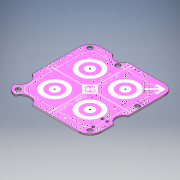
# Autodesk Inventor part: Eagle PCB rev 35
Saved by Autodesk Inventor 2016 (Build 200138000, 138)
## iProperties
Created: 2017-03-15
Part Number: Eagle PCB rev 35
Material: Generic
Document SubType Name: Modeling
Designer: Samuel Clay
Density: 1 g/cm^3
Appearance: Default
Author: Samuel Clay
Autodesk Inventor part; units mm, degrees
(part 1 of 3)
ref_plane "YZ Plane" through (0, 0, 0) normal (1, 0, 0) x (0, 1, 0)
ref_plane "XZ Plane" through (0, 0, 0) normal (0, 1, 0) x (-1, 0, 0)
ref_plane "XY Plane" through (0, 0, 0) normal (0, 0, 1) x (1, 0, 0)
sketch "PCB" plane through (0, 0, 0) normal (0, 0, 1) x (1, 0, 0)
  line L0 (18.3495, -15.3592) -> (18.2813, -15.6127)
  line L1 (15.8202, 13.2003) -> (15.9024, 13.1783)
  line L2 (15.9078, 13.2734) -> (15.9905, 13.2513)
  line L3 (-0.9735, 17.5782) -> (-0.8908, 17.6003)
  line L4 (-1.034, 17.5177) -> (-0.9735, 17.5782)
  line L5 (-1.0562, 17.435) -> (-1.034, 17.5177)
  line L6 (-1.0283, 17.4212) -> (-0.9681, 17.4814)
  line L7 (-0.8908, 17.6003) -> (-0.8082, 17.5782)
  line L8 (-0.8082, 17.5782) -> (-0.7476, 17.5177)
  line L9 (-0.7476, 17.5177) -> (-0.7255, 17.435)
  line L10 (-0.7476, 17.3523) -> (-0.8082, 17.2918)
  line L11 (-0.8082, 17.2918) -> (-0.8908, 17.2697)
  line L12 (-0.8908, 17.2697) -> (-0.9735, 17.2918)
  line L13 (-0.9735, 17.2918) -> (-1.034, 17.3523)
  line L14 (-1.034, 17.3523) -> (-1.0562, 17.435)
  line L15 (-1.034, 17.3523) -> (-1.0283, 17.4212)
  line L16 (-0.9681, 17.4814) -> (-0.8859, 17.5034)
  line L17 (-0.8859, 17.5034) -> (-0.8037, 17.4814)
  line L18 (-0.8037, 17.4814) -> (-0.7435, 17.4212)
  line L19 (-0.7435, 17.4212) -> (-0.7364, 17.3944)
  line L20 (16.6971, -16.0734) -> (16.3265, -16.444)
  line L21 (13.3467, 16.7541) -> (13.4072, 16.8146)
  line L22 (13.4072, 16.8146) -> (13.4899, 16.8368)
  line L23 (13.4899, 16.8368) -> (13.5725, 16.8146)
  line L24 (13.5725, 16.8146) -> (13.633, 16.7541)
  line L25 (13.633, 16.7541) -> (13.6552, 16.6714)
  line L26 (13.6552, 16.6714) -> (13.633, 16.5888)
  line L27 (13.633, 16.5888) -> (13.5725, 16.5282)
  line L28 (13.5725, 16.5282) -> (13.4899, 16.5061)
  line L29 (13.4899, 16.5061) -> (13.4072, 16.5282)
  line L30 (13.4072, 16.5282) -> (13.3467, 16.5888)
  line L31 (13.3467, 16.5888) -> (13.3245, 16.6714)
  line L32 (-7.6358, -7.5426) -> (-7.5426, -7.6358)
  line L33 (1.2213, 5.8377) -> (1.2815, 5.7775)
  line L34 (5.3008, 14.0051) -> (5.3599, 14.0642)
  line L35 (5.3291, 14.0816) -> (5.3896, 14.1421)
  line L36 (6.5731, 14.1102) -> (6.4904, 14.0881)
  line L37 (18.3515, -14.152) -> (17.997, -13.9776)
  line L38 (15.0616, -11.7241) -> (15.0011, -11.6636)
  line L39 (15.2875, -11.6636) -> (15.2269, -11.7241)
  line L40 (-13.5058, 2.2461) -> (-13.4453, 2.3067)
  line L41 (15.3161, -0.7795) -> (15.2556, -0.719)
  line L42 (15.1443, -11.7463) -> (15.0616, -11.7241)
  line L43 (-3.7873, -17.4275) -> (-3.8412, -17.4814)
  line L44 (-3.8412, -17.4814) -> (-3.9234, -17.5034)
  line L45 (-3.9234, -17.5034) -> (-4.0056, -17.4814)
  line L46 (-4.0056, -17.4814) -> (-4.0658, -17.4212)
  line L47 (-4.0658, -17.4212) -> (-4.0845, -17.3513)
  line L48 (13.4072, -13.633) -> (13.3467, -13.5725)
  line L49 (-4.1105, -17.435) -> (-4.0845, -17.3513)
  line L50 (-4.0845, -17.3513) -> (-4.0278, -17.2918)
  line L51 (-4.0278, -17.2918) -> (-3.9451, -17.2697)
  line L52 (-3.9451, -17.2697) -> (-3.8625, -17.2918)
  line L53 (-3.8625, -17.2918) -> (-3.802, -17.3523)
  line L54 (-3.802, -17.3523) -> (-3.7873, -17.4275)
  line L55 (-3.7873, -17.4275) -> (-3.802, -17.5177)
  line L56 (-3.802, -17.5177) -> (-3.8625, -17.5782)
  line L57 (-3.8625, -17.5782) -> (-3.9451, -17.6003)
  line L58 (-3.9451, -17.6003) -> (-4.0278, -17.5782)
  line L59 (-4.0278, -17.5782) -> (-4.0883, -17.5177)
  line L60 (-4.0883, -17.5177) -> (-4.1105, -17.435)
  line L61 (-3.0384, 1.8643) -> (-3.0162, 1.7817)
  line L62 (15.0616, -11.4377) -> (15.1443, -11.4156)
  line L63 (13.3384, 16.7234) -> (13.4156, 16.744)
  line L64 (13.4156, -13.58) -> (13.3467, -13.5725)
  line L65 (13.4899, -13.6552) -> (13.4072, -13.633)
  line L66 (13.4156, 16.744) -> (13.4978, 16.722)
  line L67 (13.4978, -13.558) -> (13.4156, -13.58)
  line L68 (13.5725, -13.633) -> (13.4899, -13.6552)
  line L69 (13.4978, 16.722) -> (13.558, 16.6618)
  line L70 (13.558, 16.6618) -> (13.58, 16.5796)
  line L71 (13.58, 16.5796) -> (13.5725, 16.5282)
  line L72 (15.2269, -11.4377) -> (15.2875, -11.4982)
  line L73 (15.2033, -11.4349) -> (15.2253, -11.5171)
  line L74 (15.2875, -11.4982) -> (15.3096, -11.5809)
  line L75 (15.2253, -11.5171) -> (15.2033, -11.5993)
  line L76 (15.3096, -11.5809) -> (15.2875, -11.6636)
  line L77 (15.2033, -11.5993) -> (15.1431, -11.6595)
  line L78 (15.1431, -11.6595) -> (15.0609, -11.6816)
  line L79 (15.2269, -11.7241) -> (15.1443, -11.7463)
  line L80 (15.0609, -11.6816) -> (15.0011, -11.6636)
  line L81 (15.0011, -11.6636) -> (14.9789, -11.5809)
  line L82 (-3.0989, 1.9249) -> (-3.0384, 1.8643)
  line L83 (14.9501, -8.815) -> (14.89, -8.8752)
  line L84 (-3.0384, 1.699) -> (-3.0989, 1.6385)
  line L85 (14.9026, -8.603) -> (14.9501, -8.6506)
  line L86 (-3.0989, 1.6385) -> (-3.1816, 1.6163)
  line L87 (-3.1816, 1.947) -> (-3.0989, 1.9249)
  line L88 (14.9501, -8.6506) -> (14.9722, -8.7328)
  line L89 (14.9722, -8.7328) -> (14.9501, -8.815)
  line L90 (-3.2642, 1.6385) -> (-3.3248, 1.699)
  line L91 (-3.3248, 1.699) -> (-3.3469, 1.7817)
  line L92 (14.89, -8.8752) -> (14.8077, -8.8972)
  line L93 (14.8077, -8.8972) -> (14.7423, -8.8797)
  line L94 (-3.3469, 1.7817) -> (-3.3248, 1.8643)
  line L95 (15.7095, -6.1193) -> (15.7315, -6.2015)
  line L96 (15.7315, -6.2015) -> (15.7095, -6.2837)
  line L97 (14.7244, -8.7811) -> (14.7466, -8.6985)
  line L98 (14.7466, -8.6985) -> (14.8071, -8.6379)
  line L99 (14.8071, -8.6379) -> (14.9026, -8.603)
  line L100 (-3.0162, 1.7817) -> (-3.0384, 1.699)
  line L101 (14.9026, -8.603) -> (14.9724, -8.6379)
  line L102 (14.9724, -8.6379) -> (15.0329, -8.6985)
  line L103 (15.0329, -8.6985) -> (15.0551, -8.7811)
  line L104 (-3.3248, 1.8643) -> (-3.2642, 1.9249)
  line L105 (15.0551, -8.7811) -> (15.0329, -8.8638)
  line L106 (15.0329, -8.8638) -> (14.9724, -8.9243)
  line L107 (14.9724, -8.9243) -> (14.8897, -8.9465)
  line L108 (14.8897, -8.9465) -> (14.8071, -8.9243)
  line L109 (14.8071, -8.9243) -> (14.7423, -8.8797)
  line L110 (-3.2642, 1.9249) -> (-3.1816, 1.947)
  line L111 (14.7423, -8.8797) -> (14.7244, -8.7811)
  line L112 (15.0987, 7.214) -> (15.0767, 7.1318)
  line L113 (15.0767, 7.2962) -> (15.0987, 7.214)
  line L114 (15.0165, 7.3564) -> (15.0767, 7.2962)
  line L115 (15.0767, 7.1318) -> (15.0253, 7.0804)
  line L116 (14.9343, 7.3785) -> (15.0165, 7.3564)
  line L117 (-3.1816, 1.6163) -> (-3.2642, 1.6385)
  line L118 (15.7095, -6.2837) -> (15.6493, -6.3439)
  line L119 (15.657, -6.0668) -> (15.7095, -6.1193)
  line L120 (15.6493, -6.3439) -> (15.5671, -6.366)
  line L121 (17.4814, -4.0943) -> (17.5034, -4.1765)
  line L122 (-13.4453, -15.0011) -> (-13.3626, -14.9789)
  line L123 (17.5034, -4.1765) -> (17.4814, -4.2588)
  line L124 (15.488, -6.2359) -> (15.5101, -6.1532)
  line L125 (15.5101, -6.1532) -> (15.5706, -6.0927)
  line L126 (15.5706, -6.0927) -> (15.657, -6.0668)
  line L127 (15.657, -6.0668) -> (15.736, -6.0927)
  line L128 (15.736, -6.0927) -> (15.7965, -6.1532)
  line L129 (15.7965, -6.1532) -> (15.8187, -6.2359)
  line L130 (15.8187, -6.2359) -> (15.7965, -6.3185)
  line L131 (15.7965, -6.3185) -> (15.736, -6.3791)
  line L132 (7.5426, -7.8903) -> (7.5085, -7.763)
  line L133 (15.736, -6.3791) -> (15.6533, -6.4012)
  line L134 (-13.2799, -15.0011) -> (-13.2194, -15.0616)
  line L135 (15.6533, -6.4012) -> (15.5671, -6.366)
  line L136 (15.5671, -6.366) -> (15.5101, -6.3185)
  line L137 (15.5101, -6.3185) -> (15.488, -6.2359)
  line L138 (-13.289, -15.2253) -> (-13.3712, -15.2033)
  line L139 (-13.3626, -15.3096) -> (-13.4453, -15.2875)
  line L140 (17.4814, -4.2588) -> (17.4212, -4.3189)
  line L141 (17.4282, -4.0411) -> (17.4814, -4.0943)
  line L142 (17.4212, -4.3189) -> (17.351, -4.3378)
  line L143 (-13.3626, -14.9789) -> (-13.2799, -15.0011)
  line L144 (-13.2194, -15.2269) -> (-13.2799, -15.2875)
  line L145 (-13.4453, -15.0011) -> (-13.5058, -15.0616)
  line L146 (17.4814, -1.7275) -> (17.4212, -1.7877)
  line L147 (17.2697, -4.1997) -> (17.2918, -4.117)
  line L148 (17.2918, -4.117) -> (17.3523, -4.0565)
  line L149 (-13.4314, -15.1431) -> (-13.4534, -15.0609)
  line L150 (17.3523, -4.0565) -> (17.4282, -4.0411)
  line L151 (-13.2799, -15.2875) -> (-13.3626, -15.3096)
  line L152 (17.4282, -4.0411) -> (17.5177, -4.0565)
  line L153 (17.5177, -4.0565) -> (17.5782, -4.117)
  line L154 (17.5782, -4.117) -> (17.6003, -4.1997)
  line L155 (17.6003, -4.1997) -> (17.5782, -4.2823)
  line L156 (17.5782, -4.2823) -> (17.5177, -4.3429)
  line L157 (17.5177, -4.3429) -> (17.435, -4.365)
  line L158 (-13.4453, -15.2875) -> (-13.5058, -15.2269)
  line L159 (17.435, -4.365) -> (17.351, -4.3378)
  line L160 (17.351, -4.3378) -> (17.2918, -4.2823)
  line L161 (17.2918, -4.2823) -> (17.2697, -4.1997)
  line L162 (1.4826, 8.3834) -> (1.3999, 8.3613)
  line L163 (-13.5058, -15.2269) -> (-13.5279, -15.1443)
  line L164 (-13.2194, -15.2269) -> (-13.289, -15.2253)
  line L165 (-13.3712, -15.2033) -> (-13.4314, -15.1431)
  line L166 (17.4212, -1.5029) -> (17.4814, -1.5631)
  line L167 (17.4814, -1.5631) -> (17.5034, -1.6453)
  line L168 (17.5034, -1.6453) -> (17.4814, -1.7275)
  line L169 (17.4212, -1.7877) -> (17.3545, -1.8056)
  line L170 (-13.4534, -15.0609) -> (-13.4453, -15.0011)
  line L171 (-13.5279, -15.1443) -> (-13.5058, -15.0616)
  line L172 (-13.2194, -15.0616) -> (-13.1972, -15.1443)
  line L173 (-13.1972, -15.1443) -> (-13.2194, -15.2269)
  line L174 (17.4212, 1.0283) -> (17.4814, 0.9681)
  line L175 (17.4814, 0.9681) -> (17.5034, 0.8859)
  line L176 (17.2697, -1.6544) -> (17.2918, -1.5717)
  line L177 (17.2918, -1.5717) -> (17.3523, -1.5112)
  line L178 (17.3523, -1.5112) -> (17.4212, -1.5029)
  line L179 (17.4212, -1.5029) -> (17.5177, -1.5112)
  line L180 (17.5177, -1.5112) -> (17.5782, -1.5717)
  line L181 (17.5782, -1.5717) -> (17.6003, -1.6544)
  line L182 (17.6003, -1.6544) -> (17.5782, -1.7371)
  line L183 (17.5782, -1.7371) -> (17.5177, -1.7976)
  line L184 (17.5177, -1.7976) -> (17.435, -1.8198)
  line L185 (17.435, -1.8198) -> (17.3545, -1.8056)
  line L186 (17.3545, -1.8056) -> (17.2918, -1.7371)
  line L187 (17.2918, -1.7371) -> (17.2697, -1.6544)
  line L188 (17.4814, 0.8037) -> (17.4212, 0.7435)
  line L189 (17.3555, 1.0459) -> (17.4212, 1.0283)
  line L190 (17.5034, 0.8859) -> (17.4814, 0.8037)
  line L191 (17.4212, 0.7435) -> (17.3944, 0.7364)
  line L192 (5.6376, 13.9989) -> (5.6155, 13.9162)
  line L193 (5.3896, 13.8557) -> (5.3291, 13.9162)
  line L194 (5.3291, 13.9162) -> (5.3008, 14.0051)
  line L195 (7.9395, -7.5937) -> (7.9734, -7.7203)
  line L196 (0.7364, 17.3944) -> (0.7435, 17.4212)
  line L197 (0.7435, 17.4212) -> (0.8037, 17.4814)
  line L198 (0.8037, 17.4814) -> (0.8859, 17.5034)
  line L199 (0.8859, 17.5034) -> (0.9681, 17.4814)
  line L200 (0.9681, 17.4814) -> (1.0283, 17.4212)
  line L201 (1.0283, 17.4212) -> (1.0459, 17.3555)
  line L202 (7.5426, -7.6358) -> (7.6358, -7.5426)
  line L203 (0.7255, 17.435) -> (0.7476, 17.5177)
  line L204 (0.7476, 17.5177) -> (0.8082, 17.5782)
  line L205 (0.8082, 17.5782) -> (0.8908, 17.6003)
  line L206 (7.763, -7.5085) -> (7.8903, -7.5426)
  line L207 (0.8908, 17.6003) -> (0.9735, 17.5782)
  line L208 (0.9735, 17.5782) -> (1.034, 17.5177)
  line L209 (1.034, 17.5177) -> (1.0562, 17.435)
  line L210 (1.0562, 17.435) -> (1.0459, 17.3555)
  line L211 (1.0459, 17.3555) -> (0.9735, 17.2918)
  line L212 (0.9735, 17.2918) -> (0.8908, 17.2697)
  line L213 (0.8908, 17.2697) -> (0.8082, 17.2918)
  line L214 (0.8082, 17.2918) -> (0.7476, 17.3523)
  line L215 (7.9395, -7.8468) -> (7.8468, -7.9395)
  line L216 (7.6358, -7.5426) -> (7.763, -7.5085)
  line L217 (-8.0556, 15.2033) -> (-7.9734, 15.2253)
  line L218 (-8.1002, 15.2875) -> (-8.0176, 15.3096)
  line L219 (12.672, 13.1181) -> (12.6941, 13.0359)
  line L220 (12.7422, 13.1907) -> (12.7644, 13.1081)
  line L221 (17.2918, 6.8276) -> (17.3523, 6.8881)
  line L222 (16.6541, -8.2122) -> (16.8879, -7.8911)
  line L223 (16.1527, -9.2892) -> (16.2848, -8.9145)
  line L224 (-3.5253, -2.1635) -> (-3.5474, -2.2461)
  line L225 (18.2813, -15.6127) -> (18.1967, -15.8611)
  line L226 (12.6817, 13.2513) -> (12.7422, 13.1907)
  line L227 (-7.8912, 15.2033) -> (-7.8422, 15.1543)
  line L228 (-7.8422, 15.1543) -> (-7.8744, 15.2269)
  line L229 (-7.9349, 15.2875) -> (-7.8744, 15.2269)
  line L230 (-1.5112, -17.3523) -> (-1.4891, -17.435)
  line L231 (18.096, -16.1034) -> (17.9797, -16.3387)
  line L232 (-3.8338, -2.0808) -> (-3.7733, -2.0203)
  line L233 (17.9797, -16.3387) -> (17.8483, -16.5658)
  line L234 (16.7895, -16.1624) -> (16.4169, -16.535)
  line L235 (1.3999, 16.5822) -> (1.4826, 16.5601)
  line L236 (16.0734, 11.9347) -> (16.1556, 11.9127)
  line L237 (16.1624, 12.0008) -> (16.245, 11.9786)
  line L238 (1.2567, 16.4996) -> (1.3172, 16.5601)
  line L239 (-2.4425, 13.0359) -> (-2.4205, 13.1181)
  line L240 (-2.4561, 13.1081) -> (-2.4339, 13.1907)
  line L241 (9.1788, 17.5177) -> (9.201, 17.435)
  line L242 (9.0357, 17.2697) -> (8.953, 17.2918)
  line L243 (-16.1624, -14.7716) -> (-15.6533, -14.6352)
  line L244 (9.1283, 17.4212) -> (9.1503, 17.339)
  line L245 (-13.4156, 10.5425) -> (-13.3452, 10.5237)
  line L246 (-3.6079, -2.0203) -> (-3.5474, -2.0808)
  line L247 (-7.3653, 16.4996) -> (-7.3432, 16.4169)
  line L248 (17.4429, -7.3239) -> (17.7589, -7.0832)
  line L249 (15.0261, -16.1624) -> (14.8897, -15.6533)
  line L250 (16.2848, -8.9145) -> (16.4524, -8.5544)
  line L251 (18.4531, 13.3626) -> (18.4531, -6.6988)
  line L252 (16.7775, -17.7069) -> (16.5591, -17.8524)
  line L253 (16.3317, -17.9834) -> (16.0962, -18.0993)
  line L254 (-1.811, -17.3509) -> (-1.8198, -17.435)
  line L255 (16.5591, -17.8524) -> (16.3317, -17.9834)
  line L256 (12.599, 13.2734) -> (12.6817, 13.2513)
  line L257 (-1.6611, 3.6259) -> (-1.601, 3.6861)
  line L258 (-1.6703, 3.646) -> (-1.6098, 3.7065)
  line L259 (15.0997, 7.1108) -> (15.0253, 7.0804)
  line L260 (16.2848, -12.0147) -> (16.1527, -11.6401)
  line L261 (18.0967, -6.8742) -> (18.4531, -6.6988)
  line L262 (15.1443, 16.535) -> (15.6533, 16.6714)
  line L263 (16.6541, -12.717) -> (16.4524, -12.3748)
  line L264 (17.7589, -7.0832) -> (18.0967, -6.8742)
  line L265 (-1.811, -17.3509) -> (-1.7371, -17.2918)
  line L266 (-11.4284, 12.5296) -> (-11.4064, 12.6118)
  line L267 (12.7422, 13.0254) -> (12.6817, 12.9649)
  line L268 (16.8879, -13.0381) -> (16.6541, -12.717)
  line L269 (-1.5112, -17.5177) -> (-1.5717, -17.5782)
  line L270 (15.6533, 16.6714) -> (16.1624, 16.535)
  line L271 (17.1517, -13.3351) -> (16.8879, -13.0381)
  line L272 (12.4337, 13.1081) -> (12.4558, 13.1907)
  line L273 (16.1527, -11.6401) -> (16.0575, -11.2544)
  line L274 (16.1624, 16.535) -> (16.535, 16.1624)
  line L275 (16.4524, -12.3748) -> (16.2848, -12.0147)
  line L276 (18.1967, -15.8611) -> (18.096, -16.1034)
  line L277 (-17.6003, 8.0176) -> (-17.5782, 8.1002)
  line L278 (15.5671, 16.5796) -> (16.0734, 16.444)
  line L279 (16.9858, -17.5473) -> (16.7775, -17.7069)
  line L280 (-8.0176, 14.9789) -> (-8.1002, 15.0011)
  line L281 (17.1833, -17.3745) -> (16.9858, -17.5473)
  line L282 (12.5296, 13.2003) -> (12.6118, 13.1783)
  line L283 (17.0151, 12.8535) -> (17.0373, 12.9362)
  line L284 (17.1517, -7.5941) -> (17.4429, -7.3239)
  line L285 (17.0978, 12.9967) -> (17.1805, 13.0189)
  line L286 (16.444, 16.0734) -> (16.5796, 15.5671)
  line L287 (16.535, 16.1624) -> (16.6714, 15.6533)
  line L288 (16.0575, -9.6748) -> (16.1527, -9.2892)
  line L289 (16, -10.0678) -> (16.0575, -9.6748)
  line L290 (16.0734, 16.444) -> (16.444, 16.0734)
  line L291 (16.0575, -11.2544) -> (16, -10.8614)
  line L292 (16.4524, -8.5544) -> (16.6541, -8.2122)
  line L293 (16.8879, -7.8911) -> (17.1517, -7.5941)
  line L294 (15.9808, -10.4646) -> (16, -10.0678)
  line L295 (17.8483, -16.5658) -> (17.7023, -16.7839)
  line L296 (12.4558, 13.0254) -> (12.4337, 13.1081)
  line L297 (-11.4087, 12.4559) -> (-11.4284, 12.5296)
  line L298 (17.7023, -16.7839) -> (17.5423, -16.9919)
  line L299 (16, -10.8614) -> (15.9808, -10.4646)
  line L300 (-8.1378, 15.0609) -> (-8.1158, 15.1431)
  line L301 (-8.1829, 15.1443) -> (-8.1607, 15.2269)
  line L302 (12.599, 12.9427) -> (12.5163, 12.9649)
  line L303 (17.3691, -17.1891) -> (17.1833, -17.3745)
  line L304 (17.5423, -16.9919) -> (17.3691, -17.1891)
  line L305 (-11.264, 12.6941) -> (-11.1855, 12.673)
  line L306 (17.4429, -13.6053) -> (17.1517, -13.3351)
  line L307 (15.6533, 14.6352) -> (15.1443, 14.7716)
  line L308 (17.7589, -13.846) -> (17.4429, -13.6053)
  line L309 (18.3515, -14.152) -> (18.4531, -14.2304)
  line L310 (17.3523, 6.6017) -> (17.2918, 6.6623)
  line L311 (18.4531, -14.2304) -> (18.0967, -14.055)
  line L312 (15.8202, -16.5796) -> (15.314, -16.444)
  line L313 (15.9078, -16.6714) -> (15.3988, -16.535)
  line L314 (16.6714, 15.6533) -> (16.535, 15.1443)
  line L315 (-8.1158, 15.1431) -> (-8.0556, 15.2033)
  line L316 (-8.1607, 15.2269) -> (-8.1002, 15.2875)
  line L317 (-3.5474, -2.0808) -> (-3.5253, -2.1635)
  line L318 (18.4528, -14.5799) -> (18.4354, -14.8417)
  line L319 (16.1624, 14.7716) -> (15.6533, 14.6352)
  line L320 (18.4354, -14.8417) -> (18.4009, -15.1019)
  line L321 (17.3523, 6.8881) -> (17.4212, 6.8502)
  line L322 (17.435, 6.9103) -> (17.5177, 6.8881)
  line L323 (18.4009, -15.1019) -> (18.3495, -15.3592)
  line L324 (16.3265, -16.444) -> (15.8202, -16.5796)
  line L325 (16.4169, -16.535) -> (15.9078, -16.6714)
  line L326 (16.0962, -18.0993) -> (15.8537, -18.1995)
  line L327 (15.1443, 14.7716) -> (14.7716, 15.1443)
  line L328 (-11.3462, 12.672) -> (-11.264, 12.6941)
  line L329 (15.8537, -18.1995) -> (15.6051, -18.2836)
  line L330 (17.0373, 12.9362) -> (17.0978, 12.9967)
  line L331 (14.7716, 15.1443) -> (14.6352, 15.6533)
  line L332 (15.6051, -18.2836) -> (15.3515, -18.3513)
  line L333 (15.3515, -18.3513) -> (15.0941, -18.4022)
  line L334 (15.0941, -18.4022) -> (14.8339, -18.4362)
  line L335 (14.8339, -18.4362) -> (14.572, -18.4531)
  line L336 (14.4051, -18.3515) -> (14.4849, -18.4531)
  line L337 (14.572, -18.4531) -> (14.4849, -18.4531)
  line L338 (14.2307, -17.997) -> (14.4051, -18.3515)
  line L339 (14.3095, -18.0967) -> (14.4849, -18.4531)
  line L340 (13.8598, -17.4429) -> (14.1005, -17.7589)
  line L341 (13.5897, -17.1517) -> (13.8598, -17.4429)
  line L342 (13.2927, -16.8879) -> (13.5897, -17.1517)
  line L343 (12.9715, -16.6541) -> (13.2927, -16.8879)
  line L344 (15.7647, 13.1907) -> (15.8252, 13.2513)
  line L345 (-16.5796, -15.5671) -> (-16.444, -15.0609)
  line L346 (12.6293, -16.4524) -> (12.9715, -16.6541)
  line L347 (12.2692, -16.2848) -> (12.6293, -16.4524)
  line L348 (0.7476, 3.7733) -> (0.8082, 3.8338)
  line L349 (11.8946, -16.1527) -> (12.2692, -16.2848)
  line L350 (15.7425, 13.1081) -> (15.7647, 13.1907)
  line L351 (11.5089, -16.0575) -> (11.8946, -16.1527)
  line L352 (11.1159, -16) -> (11.5089, -16.0575)
  line L353 (-11.2437, 12.7422) -> (-11.1855, 12.673)
  line L354 (10.7191, -15.9808) -> (11.1159, -16)
  line L355 (17.5782, 6.8276) -> (17.6003, 6.7449)
  line L356 (10.3224, -16) -> (10.7191, -15.9808)
  line L357 (-11.3264, 12.7644) -> (-11.2437, 12.7422)
  line L358 (9.9293, -16.0575) -> (10.3224, -16)
  line L359 (-12.4718, 13.6552) -> (-12.3891, 13.633)
  line L360 (9.5437, -16.1527) -> (9.9293, -16.0575)
  line L361 (9.1691, -16.2848) -> (9.5437, -16.1527)
  line L362 (8.8089, -16.4524) -> (9.1691, -16.2848)
  line L363 (8.4667, -16.6541) -> (8.8089, -16.4524)
  line L364 (8.1456, -16.8879) -> (8.4667, -16.6541)
  line L365 (15.8252, 13.2513) -> (15.9078, 13.2734)
  line L366 (7.8486, -17.1517) -> (8.1456, -16.8879)
  line L367 (-3.7525, -2.0092) -> (-3.7733, -2.0203)
  line L368 (-11.4091, 12.7422) -> (-11.3264, 12.7644)
  line L369 (7.5785, -17.4429) -> (7.8486, -17.1517)
  line L370 (12.6941, 13.0359) -> (12.6817, 12.9649)
  line L371 (-15.9377, -2.4047) -> (-15.5671, -2.0341)
  line L372 (14.8738, 7.1713) -> (14.8517, 7.254)
  line L373 (17.2697, 6.7449) -> (17.2918, 6.8276)
  line L374 (7.3378, -17.7589) -> (7.5785, -17.4429)
  line L375 (7.1287, -18.0967) -> (7.3378, -17.7589)
  line L376 (6.9534, -18.4531) -> (7.1287, -18.0967)
  line L377 (17.3237, 12.9362) -> (17.3458, 12.8535)
  line L378 (6.9534, -18.4531) -> (-13.3626, -18.4531)
  line L379 (17.3523, 6.8881) -> (17.435, 6.9103)
  line L380 (15.1823, 7.254) -> (15.1602, 7.1713)
  line L381 (-3.6079, -2.3067) -> (-3.6906, -2.3288)
  line L382 (-13.3626, -18.4531) -> (-13.6955, -18.4422)
  line L383 (-7.8422, 15.1543) -> (-7.8744, 15.0616)
  line L384 (-13.6955, -18.4422) -> (-14.027, -18.4095)
  line L385 (-11.4917, 12.599) -> (-11.4696, 12.6817)
  line L386 (-14.027, -18.4095) -> (-14.3557, -18.3553)
  line L387 (-14.3557, -18.3553) -> (-14.6801, -18.2796)
  line L388 (-14.6801, -18.2796) -> (-14.9989, -18.1829)
  line L389 (-11.1855, 12.673) -> (-11.161, 12.599)
  line L390 (-14.9989, -18.1829) -> (-15.3106, -18.0656)
  line L391 (-15.3106, -18.0656) -> (-15.6141, -17.9281)
  line L392 (-11.161, 12.599) -> (-11.1832, 12.5163)
  line L393 (-15.6141, -17.9281) -> (-15.9078, -17.7711)
  line L394 (15.1602, 7.1713) -> (15.0997, 7.1108)
  line L395 (-15.9078, -17.7711) -> (-16.1907, -17.5952)
  line L396 (-11.1832, 12.5163) -> (-11.2437, 12.4558)
  line L397 (-16.1907, -17.5952) -> (-16.4615, -17.4012)
  line L398 (16.6971, -15.0609) -> (16.8327, -15.5671)
  line L399 (16.7895, -15.1443) -> (16.9259, -15.6533)
  line L400 (-16.4615, -17.4012) -> (-16.719, -17.1898)
  line L401 (17.1805, 13.0189) -> (17.2631, 12.9967)
  line L402 (-16.719, -17.1898) -> (-16.9621, -16.9621)
  line L403 (-11.2437, 12.4558) -> (-11.3264, 12.4337)
  line L404 (-16.9621, -16.9621) -> (-17.1898, -16.719)
  line L405 (-11.3264, 12.4337) -> (-11.4087, 12.4559)
  line L406 (-17.1898, -16.719) -> (-17.4012, -16.4615)
  line L407 (-7.9349, 15.0011) -> (-8.0176, 14.9789)
  line L408 (-17.4012, -16.4615) -> (-17.5952, -16.1907)
  line L409 (-17.5952, -16.1907) -> (-17.7711, -15.9078)
  line L410 (-11.4087, 12.4559) -> (-11.4696, 12.5163)
  line L411 (-17.7711, -15.9078) -> (-17.9281, -15.6141)
  line L412 (-17.9281, -15.6141) -> (-18.0656, -15.3106)
  line L413 (-11.4696, 12.5163) -> (-11.4917, 12.599)
  line L414 (-18.0656, -15.3106) -> (-18.1829, -14.9989)
  line L415 (16.8327, -15.5671) -> (16.6971, -16.0734)
  line L416 (16.9259, -15.6533) -> (16.7895, -16.1624)
  line L417 (17.2631, 12.9967) -> (17.3237, 12.9362)
  line L418 (-18.1829, -14.9989) -> (-18.2796, -14.6801)
  line L419 (-7.8744, 15.0616) -> (-7.9349, 15.0011)
  line L420 (-18.2796, -14.6801) -> (-18.3553, -14.3557)
  line L421 (-12.5544, 13.633) -> (-12.4718, 13.6552)
  line L422 (-15.0609, -16.444) -> (-15.5671, -16.5796)
  line L423 (-15.5671, -16.5796) -> (-16.0734, -16.444)
  line L424 (-18.3553, -14.3557) -> (-18.4095, -14.027)
  line L425 (15.7647, 13.1907) -> (15.8202, 13.2003)
  line L426 (-16.0734, -16.444) -> (-16.444, -16.0734)
  line L427 (-16.444, -16.0734) -> (-16.5796, -15.5671)
  line L428 (-18.4095, -14.027) -> (-18.4422, -13.6955)
  line L429 (12.6817, 12.9649) -> (12.599, 12.9427)
  line L430 (-18.4422, -13.6955) -> (-18.4531, -13.3626)
  line L431 (-18.4531, -13.3626) -> (-18.4531, -8.3763)
  line L432 (-3.6906, -1.9981) -> (-3.6079, -2.0203)
  line L433 (-18.1449, -8.2246) -> (-18.4531, -8.3763)
  line L434 (-17.8528, -8.0438) -> (-18.1449, -8.2246)
  line L435 (12.5163, 13.2513) -> (12.599, 13.2734)
  line L436 (-17.5795, -7.8357) -> (-17.8528, -8.0438)
  line L437 (-17.3276, -7.6021) -> (-17.5795, -7.8357)
  line L438 (-17.0995, -7.3452) -> (-17.3276, -7.6021)
  line L439 (-11.4064, 12.6118) -> (-11.3462, 12.672)
  line L440 (-11.4696, 12.6817) -> (-11.4091, 12.7422)
  line L441 (-16.8973, -7.0675) -> (-17.0995, -7.3452)
  line L442 (-16.7229, -6.7715) -> (-16.8973, -7.0675)
  line L443 (17.5782, 6.6623) -> (17.5177, 6.6017)
  line L444 (-16.5779, -6.4601) -> (-16.7229, -6.7715)
  line L445 (-16.4637, -6.1361) -> (-16.5779, -6.4601)
  line L446 (14.9343, 7.1108) -> (14.8738, 7.1713)
  line L447 (16.051, 13.1907) -> (16.0732, 13.1081)
  line L448 (-16.3813, -5.8026) -> (-16.4637, -6.1361)
  line L449 (-16.3316, -5.4627) -> (-16.3813, -5.8026)
  line L450 (11.8525, 17.4814) -> (11.9127, 17.4212)
  line L451 (-16.315, -5.1196) -> (-16.3316, -5.4627)
  line L452 (-16.3316, -4.7764) -> (-16.315, -5.1196)
  line L453 (12.7644, 13.1081) -> (12.7422, 13.0254)
  line L454 (-16.3813, -4.4365) -> (-16.3316, -4.7764)
  line L455 (15.9078, 12.9427) -> (15.8252, 12.9649)
  line L456 (-16.4637, -4.103) -> (-16.3813, -4.4365)
  line L457 (-16.5779, -3.779) -> (-16.4637, -4.103)
  line L458 (-16.7229, -3.4676) -> (-16.5779, -3.779)
  line L459 (15.1602, 7.3366) -> (15.1823, 7.254)
  line L460 (-16.8973, -3.1716) -> (-16.7229, -3.4676)
  line L461 (-17.0995, -2.8939) -> (-16.8973, -3.1716)
  line L462 (-17.3276, -2.6371) -> (-17.0995, -2.8939)
  line L463 (-17.5795, -2.4035) -> (-17.3276, -2.6371)
  line L464 (15.8252, 12.9649) -> (15.7647, 13.0254)
  line L465 (-17.8528, -2.1953) -> (-17.5795, -2.4035)
  line L466 (-18.1449, -2.0145) -> (-17.8528, -2.1953)
  line L467 (-18.4531, -1.8628) -> (-18.1449, -2.0145)
  line L468 (15.0997, 7.3972) -> (15.1602, 7.3366)
  line L469 (12.4558, 13.1907) -> (12.5163, 13.2513)
  line L470 (-18.4531, -1.8628) -> (-18.4531, 14.3807)
  line L471 (14.8897, -15.6533) -> (15.0261, -15.1443)
  line L472 (-18.4531, 14.3807) -> (-18.4444, 14.647)
  line L473 (15.3988, -14.7716) -> (15.9078, -14.6352)
  line L474 (-18.4444, 14.647) -> (-18.4183, 14.9122)
  line L475 (-18.4183, 14.9122) -> (-18.3748, 15.1752)
  line L476 (17.5177, 6.6017) -> (17.435, 6.5796)
  line L477 (-18.3748, 15.1752) -> (-18.3143, 15.4347)
  line L478 (-18.3143, 15.4347) -> (-18.237, 15.6897)
  line L479 (-18.237, 15.6897) -> (-18.1431, 15.9391)
  line L480 (-18.1431, 15.9391) -> (-18.0331, 16.1819)
  line L481 (-18.0331, 16.1819) -> (-17.9075, 16.4169)
  line L482 (12.6118, 13.1783) -> (12.672, 13.1181)
  line L483 (-17.9075, 16.4169) -> (-17.7668, 16.6432)
  line L484 (-17.7668, 16.6432) -> (-17.6116, 16.8598)
  line L485 (-17.6116, 16.8598) -> (-17.4425, 17.0658)
  line L486 (-1.4891, -17.435) -> (-1.5112, -17.5177)
  line L487 (-17.4425, 17.0658) -> (-17.2603, 17.2603)
  line L488 (-17.2603, 17.2603) -> (-17.0658, 17.4425)
  line L489 (15.0261, -15.1443) -> (15.3988, -14.7716)
  line L490 (17.6003, 6.7449) -> (17.5782, 6.6623)
  line L491 (-17.0658, 17.4425) -> (-16.8598, 17.6116)
  line L492 (15.9024, 13.1783) -> (15.9626, 13.1181)
  line L493 (-16.8598, 17.6116) -> (-16.6432, 17.7668)
  line L494 (-16.6432, 17.7668) -> (-16.4169, 17.9075)
  line L495 (-16.4169, 17.9075) -> (-16.1819, 18.0331)
  line L496 (-16.1819, 18.0331) -> (-15.9391, 18.1431)
  line L497 (-15.9391, 18.1431) -> (-15.6897, 18.237)
  line L498 (11.6559, 17.4492) -> (11.688, 17.4814)
  line L499 (-15.6897, 18.237) -> (-15.4347, 18.3143)
  line L500 (17.2918, 6.6623) -> (17.2697, 6.7449)
  line L501 (-15.4347, 18.3143) -> (-15.1752, 18.3749)
  line L502 (-15.1752, 18.3749) -> (-14.9122, 18.4183)
  line L503 (11.688, 17.4814) -> (11.7703, 17.5034)
  line L504 (-14.9122, 18.4183) -> (-14.647, 18.4444)
  line L505 (14.8517, 7.254) -> (14.8738, 7.3366)
  line L506 (-14.647, 18.4444) -> (-14.3807, 18.4531)
  line L507 (2.6578, 3.8347) -> (2.74, 3.8127)
  line L508 (2.6725, 3.856) -> (2.7552, 3.8338)
  line L509 (15.9078, -14.6352) -> (16.4169, -14.7716)
  line L510 (-14.3807, 18.4531) -> (1.6083, 18.4531)
  line L511 (17.435, 6.5796) -> (17.3523, 6.6017)
  line L512 (1.76, 18.1449) -> (1.6083, 18.4531)
  line L513 (15.9905, 13.2513) -> (16.051, 13.1907)
  line L514 (1.9408, 17.8528) -> (1.76, 18.1449)
  line L515 (15.017, 7.4193) -> (15.0997, 7.3972)
  line L516 (2.1489, 17.5795) -> (1.9408, 17.8528)
  line L517 (2.3825, 17.3276) -> (2.1489, 17.5795)
  line L518 (2.6394, 17.0995) -> (2.3825, 17.3276)
  line L519 (17.2918, 3.7733) -> (17.3523, 3.8338)
  line L520 (2.9171, 16.8973) -> (2.6394, 17.0995)
  line L521 (2.7552, 3.5474) -> (2.6725, 3.5253)
  line L522 (3.2131, 16.7229) -> (2.9171, 16.8973)
  line L523 (3.5245, 16.5779) -> (3.2131, 16.7229)
  line L524 (3.8485, 16.4637) -> (3.5245, 16.5779)
  line L525 (-12.6149, 13.5725) -> (-12.5544, 13.633)
  line L526 (-3.5474, -2.2461) -> (-3.6079, -2.3067)
  line L527 (4.182, 16.3813) -> (3.8485, 16.4637)
  line L528 (4.5219, 16.3316) -> (4.182, 16.3813)
  line L529 (12.5163, 12.9649) -> (12.4558, 13.0254)
  line L530 (4.865, 16.315) -> (4.5219, 16.3316)
  line L531 (-8.0176, 15.3096) -> (-7.9349, 15.2875)
  line L532 (5.2082, 16.3316) -> (4.865, 16.315)
  line L533 (14.9343, 7.3785) -> (15.017, 7.4193)
  line L534 (5.5481, 16.3813) -> (5.2082, 16.3316)
  line L535 (-3.7733, -2.3067) -> (-3.8338, -2.2461)
  line L536 (5.8816, 16.4637) -> (5.5481, 16.3813)
  line L537 (6.2056, 16.5779) -> (5.8816, 16.4637)
  line L538 (15.9626, 13.1181) -> (15.9847, 13.0359)
  line L539 (6.517, 16.7229) -> (6.2056, 16.5779)
  line L540 (6.813, 16.8973) -> (6.517, 16.7229)
  line L541 (7.0907, 17.0995) -> (6.813, 16.8973)
  line L542 (14.8738, 7.3366) -> (14.9343, 7.3785)
  line L543 (7.3475, 17.3276) -> (7.0907, 17.0995)
  line L544 (16.051, 13.0254) -> (15.9905, 12.9649)
  line L545 (7.5812, 17.5795) -> (7.3475, 17.3276)
  line L546 (7.7893, 17.8528) -> (7.5812, 17.5795)
  line L547 (7.9701, 18.1449) -> (7.7893, 17.8528)
  line L548 (8.077, 18.3515) -> (8.1218, 18.4531)
  line L549 (16.0732, 13.1081) -> (16.051, 13.0254)
  line L550 (17.5177, 6.8881) -> (17.5782, 6.8276)
  line L551 (8.1218, 18.4531) -> (13.3626, 18.4531)
  line L552 (13.3626, 18.4531) -> (13.6955, 18.4422)
  line L553 (-3.8338, -2.2461) -> (-3.856, -2.1635)
  line L554 (13.6955, 18.4422) -> (14.027, 18.4096)
  line L555 (-8.1607, 15.0616) -> (-8.1829, 15.1443)
  line L556 (14.027, 18.4096) -> (14.3557, 18.3553)
  line L557 (15.7647, 13.0254) -> (15.7425, 13.1081)
  line L558 (-16.0734, -2.9109) -> (-15.9377, -2.4047)
  line L559 (14.3557, 18.3553) -> (14.6801, 18.2796)
  line L560 (14.6801, 18.2796) -> (14.9989, 18.1829)
  line L561 (14.9989, 18.1829) -> (15.3106, 18.0656)
  line L562 (15.3106, 18.0656) -> (15.6141, 17.9281)
  line L563 (15.6141, 17.9281) -> (15.9078, 17.7711)
  line L564 (15.9078, 17.7711) -> (16.1907, 17.5952)
  line L565 (16.1907, 17.5952) -> (16.4615, 17.4012)
  line L566 (2.74, 3.8127) -> (2.8002, 3.7525)
  line L567 (2.7552, 3.8338) -> (2.8157, 3.7733)
  line L568 (16.4615, 17.4012) -> (16.719, 17.1898)
  line L569 (11.9347, 17.339) -> (11.9218, 17.2908)
  line L570 (16.719, 17.1898) -> (16.9621, 16.9621)
  line L571 (16.9621, 16.9621) -> (17.1898, 16.719)
  line L572 (17.1898, 16.719) -> (17.4012, 16.4615)
  line L573 (17.4012, 16.4615) -> (17.5952, 16.1907)
  line L574 (11.9127, 17.4212) -> (11.9347, 17.339)
  line L575 (17.5952, 16.1907) -> (17.7711, 15.9078)
  line L576 (17.7711, 15.9078) -> (17.9281, 15.6141)
  line L577 (17.9281, 15.6141) -> (18.0656, 15.3106)
  line L578 (18.0656, 15.3106) -> (18.1829, 14.9989)
  line L579 (18.1829, 14.9989) -> (18.2796, 14.6801)
  line L580 (18.2796, 14.6801) -> (18.3553, 14.3557)
  line L581 (18.3553, 14.3557) -> (18.4095, 14.027)
  line L582 (18.4095, 14.027) -> (18.4422, 13.6955)
  line L583 (-1.5717, -17.5782) -> (-1.6544, -17.6003)
  line L584 (18.4422, 13.6955) -> (18.4531, 13.3626)
  line L585 (-3.8127, -2.2338) -> (-3.8347, -2.1516)
  line L586 (16.5796, 15.5671) -> (16.444, 15.0609)
  line L587 (10.6406, 17.4464) -> (10.6755, 17.4814)
  line L588 (11.7703, 17.5034) -> (11.8525, 17.4814)
  line L589 (-7.9734, 15.2253) -> (-7.8912, 15.2033)
  line L590 (12.4558, 13.1907) -> (12.5296, 13.2003)
  line L591 (15.0609, 16.444) -> (15.5671, 16.5796)
  line L592 (-7.8903, -7.5426) -> (-7.763, -7.5085)
  line L593 (14.6352, 15.6533) -> (14.7716, 16.1624)
  line L594 (-7.9734, -7.7203) -> (-7.9395, -7.5937)
  line L595 (-8.0176, -7.763) -> (-7.9835, -7.6358)
  line L596 (-7.3432, 16.4169) -> (-7.3653, 16.3342)
  line L597 (-7.3653, 16.3342) -> (-7.4258, 16.2737)
  line L598 (10.6755, 17.4814) -> (10.7578, 17.5034)
  line L599 (-7.4258, 16.2737) -> (-7.5085, 16.2516)
  line L600 (10.7578, 17.5034) -> (10.84, 17.4814)
  line L601 (-7.5085, 16.2516) -> (-7.5912, 16.2737)
  line L602 (10.84, 17.4814) -> (10.9002, 17.4212)
  line L603 (10.9002, 17.4212) -> (10.9222, 17.339)
  line L604 (-8.1297, 15.0306) -> (-8.1378, 15.0609)
  line L605 (-10.706, 15.4815) -> (-10.6455, 15.542)
  line L606 (-7.4671, 16.4909) -> (-7.3849, 16.4689)
  line L607 (-10.7282, 15.3988) -> (-10.706, 15.4815)
  line L608 (-7.3849, 16.4689) -> (-7.3432, 16.4169)
  line L609 (-10.6455, 15.542) -> (-10.5628, 15.5641)
  line L610 (-10.647, 15.3962) -> (-10.5868, 15.4564)
  line L611 (-10.5628, 15.5641) -> (-10.4801, 15.542)
  line L612 (-10.4801, 15.542) -> (-10.4196, 15.4815)
  line L613 (-12.6371, 13.4899) -> (-12.6149, 13.5725)
  line L614 (-10.3975, 15.3988) -> (-10.4196, 15.3161)
  line L615 (-7.6096, 16.4087) -> (-7.5494, 16.4689)
  line L616 (-10.4196, 15.3161) -> (-10.4801, 15.2556)
  line L617 (-10.4801, 15.2556) -> (-10.5628, 15.2335)
  line L618 (-10.5628, 15.2335) -> (-10.6455, 15.2556)
  line L619 (-10.6455, 15.2556) -> (-10.706, 15.3161)
  line L620 (-10.706, 15.3161) -> (-10.7282, 15.3988)
  line L621 (-7.4258, 16.5601) -> (-7.3653, 16.4996)
  line L622 (-7.5085, 16.5822) -> (-7.4258, 16.5601)
  line L623 (-10.6691, 15.314) -> (-10.647, 15.3962)
  line L624 (-12.3891, 13.633) -> (-12.3286, 13.5725)
  line L625 (-10.5868, 15.4564) -> (-10.5046, 15.4784)
  line L626 (-10.5046, 15.4784) -> (-10.4224, 15.4564)
  line L627 (-7.6358, -7.9835) -> (-7.763, -8.0176)
  line L628 (-7.5085, -7.763) -> (-7.5426, -7.8903)
  line L629 (-7.6316, 16.3265) -> (-7.6096, 16.4087)
  line L630 (-7.6738, 16.4169) -> (-7.6517, 16.4996)
  line L631 (6.3168, 14.2617) -> (6.3724, 14.3173)
  line L632 (-7.7203, -7.9734) -> (-7.8468, -7.9395)
  line L633 (-7.763, -8.0176) -> (-7.8903, -7.9835)
  line L634 (-7.6517, 16.4996) -> (-7.5912, 16.5601)
  line L635 (-7.5912, 16.5601) -> (-7.5085, 16.5822)
  line L636 (6.3724, 14.3173) -> (6.4547, 14.3394)
  line L637 (2.5072, 3.6906) -> (2.5293, 3.7733)
  line L638 (-10.6455, 15.2556) -> (-10.6691, 15.314)
  line L639 (-12.5455, 13.4978) -> (-12.4853, 13.558)
  line L640 (-7.6517, 16.3342) -> (-7.6738, 16.4169)
  line L641 (-12.3286, 13.5725) -> (-12.3064, 13.4899)
  line L642 (-7.5494, 16.4689) -> (-7.4671, 16.4909)
  line L643 (-5.9837, 17.3487) -> (-5.9642, 17.4212)
  line L644 (-12.3064, 13.4899) -> (-12.3286, 13.4072)
  line L645 (-12.3286, 13.4072) -> (-12.3891, 13.3467)
  line L646 (-12.3891, 13.3467) -> (-12.4718, 13.3245)
  line L647 (-12.4718, 13.3245) -> (-12.5544, 13.3467)
  line L648 (-12.5544, 13.3467) -> (-12.6149, 13.4072)
  line L649 (-12.6149, 13.4072) -> (-12.6371, 13.4899)
  line L650 (-12.5675, 13.4156) -> (-12.5455, 13.4978)
  line L651 (-12.4853, 13.558) -> (-12.4031, 13.58)
  line L652 (0.8859, 3.8347) -> (0.9681, 3.8127)
  line L653 (-12.4031, 13.58) -> (-12.3286, 13.5725)
  line L654 (-12.5544, 13.3467) -> (-12.5675, 13.4156)
  line L655 (-7.5426, -7.6358) -> (-7.5085, -7.763)
  line L656 (-5.9642, 17.4212) -> (-5.9041, 17.4814)
  line L657 (-6.1117, 16.3308) -> (-6.0908, 16.4087)
  line L658 (-6.1467, 16.4169) -> (-6.1245, 16.4996)
  line L659 (-5.9041, 17.4814) -> (-5.8218, 17.5034)
  line L660 (-5.8218, 17.5034) -> (-5.7396, 17.4814)
  line L661 (-5.7396, 17.4814) -> (-5.691, 17.4327)
  line L662 (-5.9813, 16.5822) -> (-5.8987, 16.5601)
  line L663 (-5.8987, 16.5601) -> (-5.8382, 16.4996)
  line L664 (-6.1245, 16.4996) -> (-6.064, 16.5601)
  line L665 (-6.064, 16.5601) -> (-5.9813, 16.5822)
  line L666 (-17.5782, 8.1002) -> (-17.5177, 8.1607)
  line L667 (-17.5177, 8.1607) -> (-17.435, 8.1829)
  line L668 (-17.4814, 8.0556) -> (-17.4212, 8.1158)
  line L669 (-1.5717, -17.2918) -> (-1.5112, -17.3523)
  line L670 (-17.435, 8.1829) -> (-17.3523, 8.1607)
  line L671 (-17.2918, 8.1002) -> (-17.2697, 8.0176)
  line L672 (-17.2697, 8.0176) -> (-17.2918, 7.9349)
  line L673 (-1.6544, -17.2697) -> (-1.5717, -17.2918)
  line L674 (-17.2918, 7.9349) -> (-17.3523, 7.8744)
  line L675 (-17.3523, 7.8744) -> (-17.435, 7.8522)
  line L676 (-17.435, 7.8522) -> (-17.5177, 7.8744)
  line L677 (-17.5177, 7.8744) -> (-17.5782, 7.9349)
  line L678 (-1.7371, -17.2918) -> (-1.6544, -17.2697)
  line L679 (-17.5782, 7.9349) -> (-17.6003, 8.0176)
  line L680 (-17.5034, 7.9734) -> (-17.4814, 8.0556)
  line L681 (-1.6544, -17.6003) -> (-1.7371, -17.5782)
  line L682 (11.4091, 12.9967) -> (11.4696, 12.9362)
  line L683 (-17.4212, 8.1158) -> (-17.339, 8.1378)
  line L684 (-12.6149, 11.5363) -> (-12.5544, 11.5968)
  line L685 (-12.5466, 11.3126) -> (-12.5675, 11.3906)
  line L686 (-12.5544, 11.5968) -> (-12.4718, 11.619)
  line L687 (-12.4718, 11.619) -> (-12.3891, 11.5968)
  line L688 (-17.435, 7.8522) -> (-17.4814, 7.8912)
  line L689 (-17.4814, 7.8912) -> (-17.5034, 7.9734)
  line L690 (-12.3891, 11.5968) -> (-12.3286, 11.5363)
  line L691 (-12.3286, 11.5363) -> (-12.3064, 11.4536)
  line L692 (-12.3064, 11.4536) -> (-12.3286, 11.371)
  line L693 (-12.3286, 11.371) -> (-12.3891, 11.3105)
  line L694 (-12.3891, 11.3105) -> (-12.4718, 11.2883)
  line L695 (-1.7371, -17.5782) -> (-1.7976, -17.5177)
  line L696 (-1.7976, -17.5177) -> (-1.8198, -17.435)
  line L697 (-12.6371, 11.4536) -> (-12.6149, 11.5363)
  line L698 (-12.5675, 11.3906) -> (-12.5455, 11.4728)
  line L699 (-12.5455, 11.4728) -> (-12.4853, 11.533)
  line L700 (-5.0625, 0.1644) -> (-5.0905, 0.1653)
  line L701 (-5.0078, 0.1432) -> (-4.9473, 0.0827)
  line L702 (-11.1545, -2.3067) -> (-11.215, -2.2461)
  line L703 (11.4284, 12.7827) -> (11.409, 12.7104)
  line L704 (-4.9473, 0.0827) -> (-4.9252, 0)
  line L705 (-11.0719, -2.3288) -> (-11.1545, -2.3067)
  line L706 (-4.9252, 0) -> (-4.9473, -0.0827)
  line L707 (-4.9473, -0.0827) -> (-5.0078, -0.1432)
  line L708 (-1.4891, -17.435) -> (-1.5631, -17.4814)
  line L709 (-5.0078, -0.1432) -> (-5.0905, -0.1653)
  line L710 (-1.5631, -17.4814) -> (-1.6453, -17.5034)
  line L711 (-1.6453, -17.5034) -> (-1.7275, -17.4814)
  line L712 (-10.9287, -2.2461) -> (-10.9892, -2.3067)
  line L713 (-1.7275, -17.4814) -> (-1.7877, -17.4212)
  line L714 (-1.7877, -17.4212) -> (-1.811, -17.3509)
  line L715 (-10.9065, -2.1635) -> (-10.9287, -2.2461)
  line L716 (-5.2049, 0.0822) -> (-5.1447, 0.1424)
  line L717 (-5.2337, 0.0827) -> (-5.1732, 0.1432)
  line L718 (4.3189, -17.4212) -> (4.2588, -17.4814)
  line L719 (11.4064, 12.865) -> (11.4284, 12.7827)
  line L720 (-5.1732, -0.1432) -> (-5.2337, -0.0827)
  line L721 (-17.4814, 2.449) -> (-17.5034, 2.5312)
  line L722 (-17.5782, 2.4626) -> (-17.6003, 2.5453)
  line L723 (4.3378, -17.351) -> (4.3189, -17.4212)
  line L724 (4.2588, -17.4814) -> (4.1765, -17.5034)
  line L725 (4.1765, -17.5034) -> (4.0943, -17.4814)
  line L726 (4.0943, -17.4814) -> (4.0411, -17.4282)
  line L727 (11.3264, 12.6882) -> (11.2437, 12.7103)
  line L728 (4.0411, -17.4282) -> (4.0565, -17.3523)
  line L729 (4.0565, -17.3523) -> (4.117, -17.2918)
  line L730 (4.117, -17.2918) -> (4.1997, -17.2697)
  line L731 (11.3264, 13.0189) -> (11.4091, 12.9967)
  line L732 (4.1997, -17.2697) -> (4.2823, -17.2918)
  line L733 (4.2823, -17.2918) -> (4.3378, -17.351)
  line L734 (4.3378, -17.351) -> (4.365, -17.435)
  line L735 (4.365, -17.435) -> (4.3429, -17.5177)
  line L736 (11.1832, 12.9362) -> (11.2437, 12.9967)
  line L737 (4.3429, -17.5177) -> (4.2823, -17.5782)
  line L738 (4.2823, -17.5782) -> (4.1997, -17.6003)
  line L739 (4.1997, -17.6003) -> (4.117, -17.5782)
  line L740 (4.117, -17.5782) -> (4.0565, -17.5177)
  line L741 (4.0565, -17.5177) -> (4.0411, -17.4282)
  line L742 (11.1832, 12.7709) -> (11.161, 12.8535)
  line L743 (11.264, 12.9472) -> (11.3462, 12.9251)
  line L744 (-5.2559, 0) -> (-5.2337, 0.0827)
  line L745 (-5.2269, 0) -> (-5.2049, 0.0822)
  line L746 (11.3462, 12.9251) -> (11.4064, 12.865)
  line L747 (-1.384, 3.4807) -> (-1.4445, 3.4202)
  line L748 (-1.601, 3.6861) -> (-1.5187, 3.7082)
  line L749 (-1.6098, 3.7065) -> (-1.5272, 3.7287)
  line L750 (2.0408, -17.4212) -> (1.9806, -17.4814)
  line L751 (2.0588, -17.3541) -> (2.0408, -17.4212)
  line L752 (1.9806, -17.4814) -> (1.8984, -17.5034)
  line L753 (1.8984, -17.5034) -> (1.8162, -17.4814)
  line L754 (1.8162, -17.4814) -> (1.7567, -17.4219)
  line L755 (11.2437, 12.7103) -> (11.1832, 12.7709)
  line L756 (0.269, -17.4212) -> (0.2088, -17.4814)
  line L757 (11.409, 12.7104) -> (11.4696, 12.7709)
  line L758 (11.4917, 12.8535) -> (11.4696, 12.7709)
  line L759 (1.7567, -17.4219) -> (1.7658, -17.3523)
  line L760 (1.7658, -17.3523) -> (1.8263, -17.2918)
  line L761 (1.8263, -17.2918) -> (1.9089, -17.2697)
  line L762 (1.9089, -17.2697) -> (1.9916, -17.2918)
  line L763 (1.9916, -17.2918) -> (2.0588, -17.3541)
  line L764 (2.0588, -17.3541) -> (2.0743, -17.435)
  line L765 (2.0743, -17.435) -> (2.0521, -17.5177)
  line L766 (2.0521, -17.5177) -> (1.9916, -17.5782)
  line L767 (-16.9972, 7.0875) -> (-16.9751, 7.1697)
  line L768 (1.9916, -17.5782) -> (1.9089, -17.6003)
  line L769 (1.9089, -17.6003) -> (1.8263, -17.5782)
  line L770 (1.8263, -17.5782) -> (1.7658, -17.5177)
  line L771 (1.7658, -17.5177) -> (1.7567, -17.4219)
  line L772 (11.409, 12.7104) -> (11.3264, 12.6882)
  line L773 (2.3225, 14.8236) -> (2.4047, 14.8456)
  line L774 (2.3353, 14.9057) -> (2.418, 14.9278)
  line L775 (-15.5671, -3.7878) -> (-15.9377, -3.4172)
  line L776 (2.5471, 14.7634) -> (2.5689, 14.6819)
  line L777 (2.5689, 14.6819) -> (2.5833, 14.7625)
  line L778 (2.5612, 14.8452) -> (2.5833, 14.7625)
  line L779 (15.2556, -0.719) -> (15.2335, -0.6363)
  line L780 (2.2623, 14.7634) -> (2.3225, 14.8236)
  line L781 (2.2748, 14.8452) -> (2.3353, 14.9057)
  line L782 (-11.1533, -17.4212) -> (-11.1753, -17.339)
  line L783 (2.2748, 14.6798) -> (2.2623, 14.7634)
  line L784 (-15.062, -3.9231) -> (-15.5671, -3.7878)
  line L785 (15.3988, -0.8017) -> (15.3161, -0.7795)
  line L786 (-13.3712, -17.4814) -> (-13.4314, -17.4212)
  line L787 (-13.4453, -17.5782) -> (-13.5058, -17.5177)
  line L788 (-15.9377, -3.4172) -> (-16.0734, -2.9109)
  line L789 (-13.4536, -17.2853) -> (-13.5058, -17.3523)
  line L790 (-16.1624, -2.927) -> (-16.026, -2.418)
  line L791 (-16.026, -2.418) -> (-15.6533, -2.0453)
  line L792 (-15.1443, -1.9089) -> (-14.6352, -2.0453)
  line L793 (-14.6352, -2.0453) -> (-14.2626, -2.418)
  line L794 (2.5007, 14.9057) -> (2.5612, 14.8452)
  line L795 (-14.2626, -2.418) -> (-14.1262, -2.927)
  line L796 (-14.1262, -2.927) -> (-14.2626, -3.4361)
  line L797 (-13.2194, -17.5177) -> (-13.2799, -17.5782)
  line L798 (-14.2626, -3.4361) -> (-14.6352, -3.8087)
  line L799 (-15.1443, -3.9451) -> (-15.6533, -3.8087)
  line L800 (-15.6533, -3.8087) -> (-16.026, -3.4361)
  line L801 (-16.026, -3.4361) -> (-16.1624, -2.927)
  line L802 (-11.0109, -17.5034) -> (-11.0931, -17.4814)
  line L803 (-13.2799, -17.5782) -> (-13.3626, -17.6003)
  line L804 (15.542, -0.5536) -> (15.5641, -0.6363)
  line L805 (15.2556, -0.5536) -> (15.3161, -0.4931)
  line L806 (-13.3626, -17.6003) -> (-13.4453, -17.5782)
  line L807 (2.418, 14.9278) -> (2.5007, 14.9057)
  line L808 (-10.8944, -17.4471) -> (-10.9287, -17.4814)
  line L809 (15.4815, -0.4931) -> (15.542, -0.5536)
  line L810 (-13.5058, -17.5177) -> (-13.5279, -17.435)
  line L811 (17.5034, 3.6703) -> (17.4814, 3.5881)
  line L812 (17.4814, 3.7525) -> (17.5034, 3.6703)
  line L813 (17.4212, 3.8127) -> (17.4814, 3.7525)
  line L814 (15.2335, -0.6363) -> (15.2556, -0.5536)
  line L815 (17.4814, 3.5881) -> (17.4268, 3.5335)
  line L816 (17.3523, 3.8338) -> (17.4212, 3.8127)
  line L817 (13.5421, 15.4405) -> (13.7952, 15.3727)
  line L818 (-13.2194, -17.3523) -> (-13.1972, -17.435)
  line L819 (13.7952, 15.3727) -> (13.9805, 15.1874)
  line L820 (13.9805, 15.1874) -> (14.0484, 14.9343)
  line L821 (-11.0931, -17.4814) -> (-11.1533, -17.4212)
  line L822 (14.0484, 14.9343) -> (13.982, 14.6865)
  line L823 (13.289, 15.3727) -> (13.5421, 15.4405)
  line L824 (-14.4439, 9.4099) -> (-14.4659, 9.4921)
  line L825 (17.5034, 6.7078) -> (17.4814, 6.6256)
  line L826 (13.1081, 15.017) -> (13.1763, 15.2715)
  line L827 (13.3626, 15.4579) -> (13.6171, 15.5261)
  line L828 (15.4815, -0.7795) -> (15.3988, -0.8017)
  line L829 (13.6171, 15.5261) -> (13.8716, 15.4579)
  line L830 (13.8716, 15.4579) -> (14.058, 15.2715)
  line L831 (8.0692, 16.2279) -> (8.2265, 16.3852)
  line L832 (14.058, 15.2715) -> (14.1262, 15.017)
  line L833 (14.1262, 15.017) -> (14.058, 14.7625)
  line L834 (2.5689, 14.6819) -> (2.5007, 14.6193)
  line L835 (13.8716, 14.5762) -> (13.6171, 14.508)
  line L836 (-13.5279, -17.435) -> (-13.5058, -17.3523)
  line L837 (2.4869, 14.8236) -> (2.5471, 14.7634)
  line L838 (13.6171, 14.508) -> (13.3626, 14.5762)
  line L839 (13.3626, 14.5762) -> (13.1763, 14.7625)
  line L840 (13.1763, 14.7625) -> (13.1081, 15.017)
  line L841 (-10.9287, -17.4814) -> (-11.0109, -17.5034)
  line L842 (-13.2799, -17.2918) -> (-13.2194, -17.3523)
  line L843 (-13.4536, -17.2853) -> (-13.3626, -17.2697)
  line L844 (15.3161, -0.4931) -> (15.3988, -0.471)
  line L845 (8.4796, 16.453) -> (8.7328, 16.3852)
  line L846 (15.5641, -0.6363) -> (15.542, -0.719)
  line L847 (-4.8094, -14.4659) -> (-4.8916, -14.4439)
  line L848 (-13.3626, -17.2697) -> (-13.2799, -17.2918)
  line L849 (13.982, 14.6865) -> (14.058, 14.7625)
  line L850 (-11.1753, -17.339) -> (-11.1621, -17.2898)
  line L851 (2.418, 14.5971) -> (2.3353, 14.6193)
  line L852 (15.3988, -0.471) -> (15.4815, -0.4931)
  line L853 (-14.3015, 9.6566) -> (-14.2345, 9.6386)
  line L854 (8.7328, 16.3852) -> (8.9181, 16.1999)
  line L855 (8.9181, 16.1999) -> (8.9859, 15.9468)
  line L856 (2.4047, 14.8456) -> (2.4869, 14.8236)
  line L857 (8.9859, 15.9468) -> (8.9318, 15.7449)
  line L858 (-13.289, -17.5034) -> (-13.3712, -17.4814)
  line L859 (8.2265, 16.3852) -> (8.4796, 16.453)
  line L860 (2.2623, 14.7634) -> (2.2748, 14.8452)
  line L861 (17.4814, 6.6256) -> (17.435, 6.5796)
  line L862 (17.4212, 6.8502) -> (17.4814, 6.79)
  line L863 (17.4814, 6.79) -> (17.5034, 6.7078)
  line L864 (2.5007, 14.6193) -> (2.418, 14.5971)
  line L865 (-14.3837, 9.6345) -> (-14.3015, 9.6566)
  line L866 (8.0858, 16.2896) -> (8.2721, 16.476)
  line L867 (-13.4453, 2.3067) -> (-13.3626, 2.3288)
  line L868 (-13.2099, -17.4822) -> (-13.289, -17.5034)
  line L869 (8.2721, 16.476) -> (8.5266, 16.5442)
  line L870 (8.5266, 16.5442) -> (8.7811, 16.476)
  line L871 (8.7811, 16.476) -> (8.9675, 16.2896)
  line L872 (8.9675, 16.2896) -> (9.0357, 16.0351)
  line L873 (9.0357, 16.0351) -> (8.9675, 15.7806)
  line L874 (-13.4534, -17.339) -> (-13.4536, -17.2853)
  line L875 (8.7811, 15.5943) -> (8.5266, 15.5261)
  line L876 (8.5266, 15.5261) -> (8.2721, 15.5943)
  line L877 (8.2721, 15.5943) -> (8.0858, 15.7806)
  line L878 (8.0858, 15.7806) -> (8.0176, 16.0351)
  line L879 (-13.4314, -17.4212) -> (-13.4534, -17.339)
  line L880 (2.3353, 14.6193) -> (2.2748, 14.6798)
  line L881 (-14.546, 9.5447) -> (-14.5239, 9.6274)
  line L882 (-14.5239, 9.6274) -> (-14.4634, 9.6879)
  line L883 (-14.4634, 9.6879) -> (-14.3807, 9.71)
  line L884 (-14.4439, 9.5744) -> (-14.3837, 9.6345)
  line L885 (-14.3807, 9.71) -> (-14.298, 9.6879)
  line L886 (-14.298, 9.6879) -> (-14.2345, 9.6386)
  line L887 (-14.2345, 9.6386) -> (-14.2154, 9.5447)
  line L888 (-14.2154, 9.5447) -> (-14.2375, 9.462)
  line L889 (-14.2375, 9.462) -> (-14.298, 9.4015)
  line L890 (-14.298, 9.4015) -> (-14.3807, 9.3794)
  line L891 (-14.4634, 9.4015) -> (-14.5239, 9.462)
  line L892 (-14.5239, 9.462) -> (-14.546, 9.5447)
  line L893 (-14.4659, 9.4921) -> (-14.4439, 9.5744)
  line L894 (-12.7644, 3.0543) -> (-12.7422, 3.137)
  line L895 (-12.7422, 3.137) -> (-12.6817, 3.1975)
  line L896 (-12.6817, 3.1975) -> (-12.599, 3.2196)
  line L897 (-12.672, 3.1197) -> (-12.6118, 3.1799)
  line L898 (-12.5296, 3.2019) -> (-12.599, 3.2196)
  line L899 (-12.5296, 3.2019) -> (-12.4558, 3.137)
  line L900 (-12.4558, 3.137) -> (-12.4337, 3.0543)
  line L901 (-12.4337, 3.0543) -> (-12.4558, 2.9716)
  line L902 (-12.4558, 2.9716) -> (-12.5163, 2.9111)
  line L903 (-12.5163, 2.9111) -> (-12.599, 2.889)
  line L904 (-12.599, 2.889) -> (-12.6817, 2.9111)
  line L905 (-12.6817, 2.9111) -> (-12.7422, 2.9716)
  line L906 (-12.7422, 2.9716) -> (-12.7644, 3.0543)
  line L907 (-12.6941, 3.0375) -> (-12.672, 3.1197)
  line L908 (-12.6118, 3.1799) -> (-12.5296, 3.2019)
  line L909 (-12.599, 2.889) -> (-12.672, 2.9553)
  line L910 (-12.672, 2.9553) -> (-12.6941, 3.0375)
  line L911 (-17.5034, -0.7594) -> (-17.4814, -0.6772)
  line L912 (-17.4814, -0.6772) -> (-17.4212, -0.617)
  line L913 (-17.4212, -0.617) -> (-17.3931, -0.6095)
  line L914 (-4.8916, -14.4439) -> (-4.9518, -14.3837)
  line L915 (-4.9518, -14.3837) -> (-4.9738, -14.3015)
  line L916 (-4.6673, -14.384) -> (-4.7271, -14.4439)
  line L917 (-4.7271, -14.4439) -> (-4.8094, -14.4659)
  line L918 (-5.0013, -14.3807) -> (-4.9738, -14.3015)
  line L919 (-4.9738, -14.3015) -> (-4.9187, -14.2375)
  line L920 (-4.9187, -14.2375) -> (-4.836, -14.2154)
  line L921 (-4.836, -14.2154) -> (-4.7533, -14.2375)
  line L922 (-4.7533, -14.2375) -> (-4.6928, -14.298)
  line L923 (-4.6928, -14.298) -> (-4.6673, -14.384)
  line L924 (-4.6673, -14.384) -> (-4.6928, -14.4634)
  line L925 (-4.6928, -14.4634) -> (-4.7533, -14.5239)
  line L926 (-4.7533, -14.5239) -> (-4.836, -14.546)
  line L927 (-4.836, -14.546) -> (-4.9187, -14.5239)
  line L928 (-4.9187, -14.5239) -> (-4.9792, -14.4634)
  line L929 (-4.9792, -14.4634) -> (-5.0013, -14.3807)
  line L930 (14.2397, 13.4369) -> (14.3015, 13.4534)
  line L931 (14.3015, 13.4534) -> (14.3837, 13.4314)
  line L932 (14.3837, 13.4314) -> (14.4439, 13.3712)